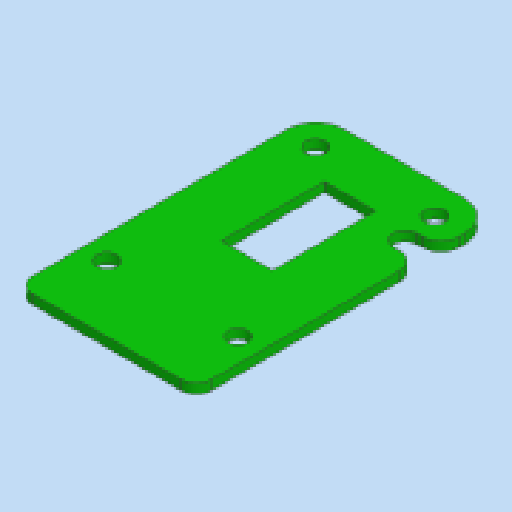
# Autodesk Inventor part: sensor_pcb
Saved by Autodesk Inventor 2024 (Build 280153000, 153)
## iProperties
Created: 2025-05-06
Part Number: sensor_pcb
Material: Generic
Document SubType Name: Modeling
Designer: XxPan
Density: 1 g/cm^3
Appearance: Default
Author: XxPan
Autodesk Inventor part; units mm, degrees
ref_plane "YZ Plane" through (0, 0, 0) normal (1, 0, 0) x (0, 1, 0)
ref_plane "XZ Plane" through (0, 0, 0) normal (0, 1, 0) x (-1, 0, 0)
ref_plane "XY Plane" through (0, 0, 0) normal (0, 0, 1) x (1, 0, 0)
sketch "Sketch1" plane through (0, 0, 0) normal (0, 1, 0) x (-1, 0, 0)
  line L0 (12.5, 32) -> (-12.5, 32)
  line L1 (-10, -18) -> (10, -18)
  line L2 (15, -13) -> (15, 29.5)
  line L3 (22.4497, 0) -> (-22.4497, 0) construction
  line L4 (0, -29.3462) -> (0, 42.8284) construction
  arc A0 (-15, -13) -> (-10, -18) centre (-10, -13) ccw
  arc A1 (10, -18) -> (15, -13) centre (10, -13) ccw
  arc A2 (-12.5, 32) -> (-15, 29.5) centre (-12.5, 29.5) ccw
  arc A3 (15, 29.5) -> (12.5, 32) centre (12.5, 29.5) ccw
  line L5 (-12, -9) -> (-9, -9)
  line L6 (-9, -9) -> (-9, -5)
  line L7 (-9, -5) -> (-12, -5)
  line L8 (-15, 29.5) -> (-15, -2)
  line L9 (-15, -12) -> (-15, -13)
  arc A4 (-15, -2) -> (-12, -5) centre (-12, -2) ccw
  arc A5 (-12, -9) -> (-15, -12) centre (-12, -12) ccw
  point P0 (0, 0)
  point P1 (15, 32)
  point P2 (-15, -18)
  point P3 (-15, 32)
  point P4 (15, -18)
  point P5 (-9, -7)
  dimension "d4" = 18
  dimension "d5" = 32
  dimension "d6" = 15
  dimension "d10" = 5
  dimension "d11" = 2.5
  dimension "d12" = 4
  dimension "d13" = 4
  dimension "d15" = 15
  dimension "d16" = 6
  dimension "d17" = 3
  constraints: 16 end point, 14 tangent, 12 point on circle, 6 centre point, 6 point on line, 5 perpendicular, 3 equal radius, 3 parallel, 2 horizontal, 1 midpoint
  measures "d4" distance between parallel lines of L1 L3
  measures "d5" distance between parallel lines of L0 L3
  measures "d6" distance between parallel lines of L4 L2
  measures "d10" radius of A0
  measures "d11" radius of A2
  measures "d12" distance from line of L9.end L5
  measures "d13" distance between parallel lines of L7 L5
  measures "d15" distance between parallel lines of L4 L9
  measures "d16" distance from line of L8 point (-9, -7)
  measures "d17" radius of A4
extrude "Extrusion1" add sketch "Sketch1" along normal blind 1.6
fillet "Fillet3" radius 2 2 edges at (9, 0.8, -5) (9, 0.8, -9)
sketch "Sketch2" plane through (0, 1.6, 0) normal (0, 1, 0) x (1, 0, 0)
  line L0 (15, 12) -> (15, 13) projected
  arc A0 (15, 13) -> (10, 18) centre (10, 13) ccw projected
  arc A1 (-10, 18) -> (-15, 13) centre (-10, 13) ccw projected
  line L1 (-15, 13) -> (-15, -29.5) projected
  line L2 (15, -29.5) -> (15, 2) projected
  line L3 (-12.5, -32) -> (12.5, -32) projected
  point P0 (0, 0)
  point P1 (-11, -21)
  point P2 (11, -21)
  dimension "d27" = 4
  dimension "d28" = 4
  dimension "d34" = 11
  constraints: 2 coincident, 2 horizontal alignment
  measures "d27" distance from line of L1 point (-11, -21)
  measures "d28" distance from line of L2 point (11, -21)
  measures "d34" distance from line of L3 point (11, -21)
hole "Hole1" at (10, 1.6, -13) at (-10, 1.6, -13) at (-11, 1.6, 21) at (11, 1.6, 21) direction (0, -1, 0) diameter 3.4 end through all
sketch "Sketch3" plane through (0, 1.6, 0) normal (0, 1, 0) x (1, 0, 0)
  line L0 (4.3, -8.51) -> (-4.3, -8.51)
  line L1 (-4.3, -8.51) -> (-4.3, 8.75)
  line L2 (-4.3, 8.75) -> (4.3, 8.75)
  line L3 (4.3, 8.75) -> (4.3, -8.51)
  line L4 (0, 28) -> (0, -42) construction
  line L5 (10, 18) -> (-10, 18) projected
  point P0 (0, 0)
  dimension "d29" = 9.25
  dimension "d30" = 8.6
  dimension "d31" = 17.26
  constraints: 8 end point, 2 parallel, 1 horizontal, 1 perpendicular, 1 other
  measures "d29" distance between parallel lines of L5 L2
  measures "d30" distance of L1.end L2.end
  measures "d31" distance of L0.end L1.end
extrude "Extrusion2" cut sketch "Sketch3" against normal through all
body "Solid1"
